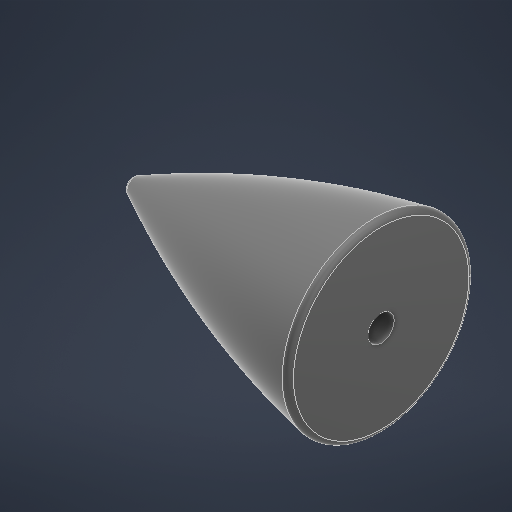
# Autodesk Inventor part: P_MotorNose
Saved by Autodesk Inventor 2026 (Build 300175000, 175)
## iProperties
Created: 2025-08-24
Part Number: P_MotorNose
Material: ABS-Kunststoff
Document SubType Name: Modeling
Designer: FAL
Density: 1.06 g/cm^3
Appearance: Glatt - Weiß
Mass: 22.3396 g
Surface Area: 46.4279 cm^2
Volume: 21.0751 cm^3
Author: FAL
Autodesk Inventor part; units mm, degrees
ref_plane "YZ Plane" through (0, 0, 0) normal (1, 0, 0) x (0, 1, 0)
ref_plane "XZ Plane" through (0, 0, 0) normal (0, 1, 0) x (-1, 0, 0)
ref_plane "XY Plane" through (0, 0, 0) normal (0, 0, 1) x (1, 0, 0)
sketch "Skizze1" plane through (0, 0, 0) normal (0, 0, 1) x (1, 0, 0)
  line L0 (0, 0) -> (-48, 0)
  line L1 (-24.1554, 13.7426) -> (0, 18) construction
  spline S0 degree 2 poles (-48, 1.1812) (-24.1554, 13.7426) (0, 18) knots 1.032137 1.032137 1.032137 2 2 2
  line L2 (0, 18) -> (0, 0)
  line L3 (-48, 0) -> (-48, 1.1812)
  line L4 (-48, 1.1812) -> (-24.1554, 13.7426) construction
  dimension "d1" = 18
  dimension "d2" = 48
  constraints: 7 end point, 2 vertical, 1 horizontal, 3 other
  measures "d1" distance of L1.end L0.start
  measures "d2" distance between parallel lines of L2 L3
revolve "Umdrehung1" add sketch "Skizze1" angle 360 about axis through (0, 0, 0) along (-1, 0, 0)
fillet "Rundung1" radius 1.5 1 edges at (-48, -1.1812, 0)
sketch "Skizze2" plane through (0, 0, 0) normal (1, 0, 0) x (0, 0, -1)
  circle A0 centre (0, 0) radius 2.5
  dimension "d4" = 5
  constraints: 1 centre point, 1 coincident
  measures "d4" diameter of A0
extrude "Extrusion1" cut sketch "Skizze2" against normal blind 17.5
fillet "Rundung2" radius 1 1 edges at (0, -18, 0)
